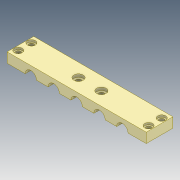
# Autodesk Inventor part: cylinder-holder-1
Saved by Autodesk Inventor 2017 (Build 210142000, 142)
## iProperties
Created: 2018-06-17
Part Number: cylinder-holder-1
Material: Nylon 6/6
Document SubType Name: Modeling
Designer: Luiz Gustavo
Density: 1.13 g/cm^3
Appearance: Nylon 6
Mass: 33.1431 g
Surface Area: 117.541 cm^2
Volume: 29.3301 cm^3
Author: Luiz Gustavo
Autodesk Inventor part; units mm, degrees
ref_plane "YZ Plane" through (0, 0, 0) normal (1, 0, 0) x (0, 1, 0)
ref_plane "XZ Plane" through (0, 0, 0) normal (0, 1, 0) x (-1, 0, 0)
ref_plane "XY Plane" through (0, 0, 0) normal (0, 0, 1) x (1, 0, 0)
sketch "Sketch1" plane through (0, 0, 0) normal (0, 0, 1) x (1, 0, 0)
  line L0 (18.1, 0) -> (18.1, 27) projected
  line L1 (18.1, 27) -> (-0.25, 27) projected
  line L2 (0, 0) -> (18.1, 0)
  circle A0 centre (13.6, 6.8375) radius 2.5 projected
  circle A1 centre (13.6, 20.1625) radius 2.5 projected
  line L3 (-104.55, 27) -> (-122.9, 27) projected
  line L4 (-122.9, 0) -> (-122.9, 27) projected
  line L5 (-104.55, 0) -> (-122.9, 0) projected
  circle A2 centre (-118.4, 6.8375) radius 2.5 projected
  circle A3 centre (-118.4, 20.1625) radius 2.5 projected
  line L6 (-104.55, 27) -> (-0.25, 27)
  line L7 (-104.55, 0) -> (0, 0)
  constraints: 6 end point, 1 collinear, 1 horizontal
extrude "Extrusion1" add sketch "Sketch1" along normal blind 10
hole "Hole1" at (13.6, 20.1625, 10) direction (0, 0, -1) diameter 8 depth 2
hole "Hole2" at (13.6, 6.8375, 10) direction (0, 0, -1) diameter 8 depth 2
hole "Hole3" at (-118.4, 20.1625, 10) direction (0, 0, -1) diameter 8 depth 2
hole "Hole4" at (-118.4, 6.8375, 10) direction (0, 0, -1) diameter 8 depth 2
chamfer "Chamfer1" [suppressed]
sketch "Sketch2" plane through (0, 0, 0) normal (0, 1, 0) x (-1, 0, 0)
  line L0 (-18.1, 0) -> (104.6, 0) construction
  circle A0 centre (6.05, 0) radius 5.75
  circle A1 centre (29.25, 0) radius 5.75
  circle A2 centre (52.45, 0) radius 5.75
  circle A3 centre (29.25, 0) radius 5.75
  circle A4 centre (75.65, 0) radius 5.75
  circle A5 centre (98.85, 0) radius 5.75
  line L1 (-18.1, 0) -> (0, 0) construction
  line L2 (122.9, 0) -> (122.9, 10) projected
  line L3 (122.9, 0) -> (122.9, 10) projected
  line L4 (-18.1, 0) -> (-18.1, 10) projected
  line L5 (-18.1, 0) -> (-18.1, 10) projected
  dimension "d49" = 11.5
  dimension "d50" = 23.2
  dimension "d51" = 23.2
  dimension "d52" = 23.2
  dimension "d54" = 23.2
  dimension "d55" = 23.2
  constraints: 6 point on line, 5 centre point, 4 end point, 4 equal radius, 2 horizontal, 1 coincident, 1 collinear, 1 horizontal alignment, 3 other
  measures "d49" diameter of A0
  measures "d50" distance of A1.centre A0.centre
  measures "d51" distance of A2.centre A1.centre
  measures "d52" distance of A2.centre A3.centre
  measures "d54" distance of A4.centre A2.centre
  measures "d55" distance of A4.centre point (98.85, 0)
extrude "Extrusion2" cut sketch "Sketch2" along normal through all
sketch "Sketch3" plane through (0, 0, 0) normal (0, 0, 1) x (1, 0, 0)
  line L0 (-69.9, 0) -> (-69.9, 27) projected
  line L1 (-58.2, 27) -> (-69.9, 27) projected
  line L2 (-58.2, 27) -> (-58.2, 0) projected
  line L3 (-69.9, 0) -> (-58.2, 0) projected
  line L4 (-35, 27) -> (-35, 0) projected
  line L5 (-46.7, 0) -> (-35, 0) projected
  line L6 (-46.7, 0) -> (-46.7, 27) projected
  line L7 (-35, 27) -> (-46.7, 27) projected
  circle A0 centre (-64.05, 13.5) radius 2.6
  circle A1 centre (-40.85, 13.5) radius 2.6
  line L8 (-69.9, 0) -> (-69.9, 27) projected
  line L9 (-69.9, 13.5) -> (-35, 13.5) construction
  line L10 (-64.05, 0) -> (-64.05, 27) construction
  line L11 (-122.9, 0) -> (18.1, 0) projected
  line L12 (-40.85, 0) -> (-40.85, 27) construction
  point P0 (0, 0)
  point P1 (-40.85, 13.5)
  dimension "d66" = 5.2
  constraints: 7 midpoint, 6 end point, 2 centre point, 2 coincident, 1 equal radius, 1 point on line
  measures "d66" diameter of A0
extrude "Extrusion3" cut sketch "Sketch3" along normal through all contours A0 | A1
hole "Hole5" at (-40.85, 13.5, 10) direction (0, 0, -1) diameter 9.5 depth 3
hole "Hole6" at (-64.05, 13.5, 10) direction (0, 0, -1) diameter 9.5 depth 3
equation "\"d51\" = d50"
equation "\"d52\" = d50"
equation "\"d54\" = d50"
equation "\"d55\" = d50"
body "Solid1"
